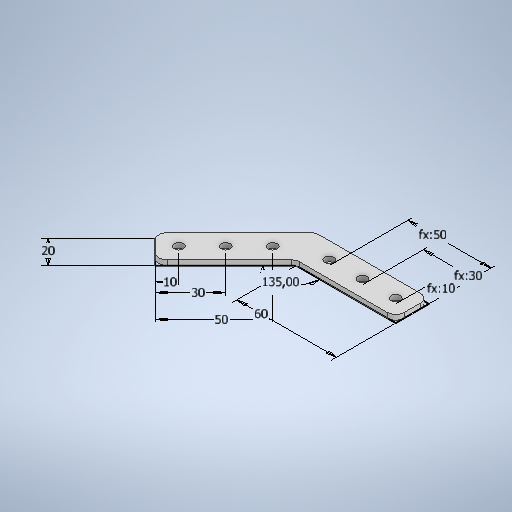
# Autodesk Inventor part: Verbinder_45deg
Saved by Autodesk Inventor 2025.1 (Build 291241000, 241)
## iProperties
Created: 2024-10-14
Part Number: Verbinder_45deg
Material: Generisch
Document SubType Name: Modeling
Designer: Kai Altwicker
Density: 1 g/cm^3
Appearance: Vorgabe
Author: Kai Altwicker
Autodesk Inventor part; units mm, degrees
ref_plane "YZ Plane" through (0, 0, 0) normal (1, 0, 0) x (0, 1, 0)
ref_plane "XZ Plane" through (0, 0, 0) normal (0, 1, 0) x (-1, 0, 0)
ref_plane "XY Plane" through (0, 0, 0) normal (0, 0, 1) x (1, 0, 0)
sketch "Skizze1" plane through (0, 0, 0) normal (0, 1, 0) x (-1, 0, 0)
  line L0 (-68.2843, 0) -> (0, 0)
  line L1 (0, 0) -> (48.2843, 48.2843)
  line L2 (48.2843, 48.2843) -> (34.1421, 62.4264)
  line L3 (34.1421, 62.4264) -> (-8.2843, 20)
  line L4 (-8.2843, 20) -> (-68.2843, 20)
  line L5 (-68.2843, 20) -> (-68.2843, 0)
  line L6 (-68.2843, 10) -> (-4.1421, 10) construction
  line L7 (-4.1421, 10) -> (41.2132, 55.3553) construction
  point P0 (-58.2843, 10)
  point P1 (-38.2843, 10)
  point P2 (-18.2843, 10)
  point P3 (5.8579, 20)
  point P4 (34.1421, 48.2843)
  point P5 (20, 34.1421)
  dimension "d3" = 60
  dimension "d4" = 20
  dimension "d5" = 135
  dimension "d6" = 10
  dimension "d7" = 30
  dimension "d8" = 50
  dimension "d9" = 10
  dimension "d10" = 30
  dimension "d11" = 50
  constraints: 17 end point, 6 point on line, 4 parallel, 2 equal length, 2 midpoint, 2 perpendicular, 1 coincident, 1 vertical
  measures "d3" distance of L3.end L4.end
  measures "d4" distance of L1.end L2.end
  measures "d5" angle of L4 L3
  measures "d6" distance from line of L2 point (34.142, 48.284)
  measures "d7" distance from line of L2 point (20, 34.142)
  measures "d8" distance from line of L2 point (5.858, 20)
  measures "d9" distance from line of L5 point (-58.284, 10)
  measures "d10" distance from line of L5 point (-38.284, 10)
  measures "d11" distance from line of L5 point (-18.284, 10)
extrude "Extrusion1" add sketch "Skizze1" along normal blind 3
fillet "Rundung1" radius 5 6 edges at (-34.1421, 1.5, 62.4264) (-48.2843, 1.5, 48.2843) (8.2843, 1.5, 20) (0, 1.5, 0) (68.2843, 1.5, 20) (68.2843, 1.5, 0)
hole "Bohrung1" at (58.2843, 0, 10) at (38.2843, 0, 10) at (18.2843, 0, 10) at (-5.8579, 0, 20) at (-34.1421, 0, 48.2843) at (-20, 0, 34.1421) direction (0, 1, 0) diameter 5.5 end through all clearance for "Flachkopfsenkschraube DIN EN ISO 2009" size "M5" standard "DIN"
equation "\"d9\" = d6"
equation "\"d10\" = d7"
equation "\"d11\" = d8"
equation "\"d_tol\" = 0.3"
equation "\"d_wand\" = 1.5"
equation "\"D_oct\" = 3573.03607"
equation "\"d_traeger\" = 625"
